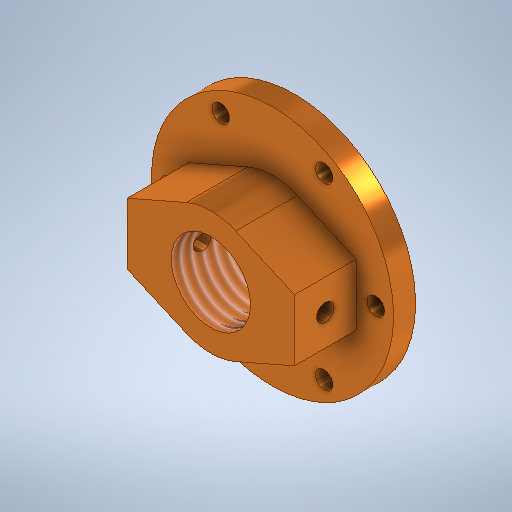
# Autodesk Inventor part: 109
Saved by Autodesk Inventor 2025.1 (Build 291241000, 241)
## iProperties
Created: 2024-06-07
Part Number: 109
Material: Gold
Document SubType Name: Modeling
Designer: ffogue
Density: 19.3 g/cm^3
Appearance: Metall - 1600F (heiß)
Author: ffogue
Autodesk Inventor part; units mm, degrees
ref_plane "YZ Plane" through (0, 0, 0) normal (1, 0, 0) x (0, 1, 0)
ref_plane "XZ Plane" through (0, 0, 0) normal (0, 1, 0) x (-1, 0, 0)
ref_plane "XY Plane" through (0, 0, 0) normal (0, 0, 1) x (1, 0, 0)
sketch "Skizze1" plane through (0, 0, 0) normal (0, 1, 0) x (-1, 0, 0)
  circle A0 centre (0, 0) radius 27.5
  dimension "d0" = 55
  constraints: 1 centre point, 1 coincident
  measures "d0" diameter of A0
extrude "Extrusion1" add sketch "Skizze1" along normal blind 5
sketch "Skizze2" plane through (0, 5, 0) normal (0, 1, 0) x (1, 0, 0)
  circle A0 centre (0, 0) radius 15
  dimension "d4" = 30
  constraints: 1 centre point, 1 coincident
  measures "d4" diameter of A0
extrude "Extrusion2" add sketch "Skizze2" along normal blind 1.5
sketch "Skizze3" plane through (0, 6.5, 0) normal (0, 1, 0) x (1, 0, 0)
  circle A0 centre (0, 0) radius 15 projected
  line L0 (-6.5, 13.5185) -> (-6.5, 12)
  line L1 (-4.5, 10) -> (4.5, 10)
  line L2 (6.5, 12) -> (6.5, 13.5185)
  line L3 (0, -15) -> (0, 15) construction
  arc A1 (-6.5, 12) -> (-4.5, 10) centre (-4.5, 12) ccw
  arc A2 (4.5, 10) -> (6.5, 12) centre (4.5, 12) ccw
  point P0 (-6.5, 10)
  point P1 (6.5, 10)
  dimension "d7" = 13
  dimension "d8" = 10
  dimension "d9" = 2
  constraints: 8 end point, 8 point on circle, 4 point on line, 4 tangent, 2 centre point, 2 perpendicular, 2 vertical, 1 equal radius, 1 horizontal alignment, 1 midpoint, 1 other
  measures "d7" distance of point (-6.5, 10) point (6.5, 10)
  measures "d8" distance from line of L1 point (0, 0)
  measures "d9" radius of A1
extrude "Extrusion3" cut sketch "Skizze3" against normal blind 1.5 contours L2 A2 L1 A1 L0 A0 picked at (0, 11.6667)
sketch "Skizze4" plane through (0, 5, 0) normal (0, 1, 0) x (1, 0, 0)
  circle A0 centre (0, 0) radius 23.5 construction
  point P0 (-23.5, 0)
  dimension "d12" = 47
  constraints: 2 horizontal alignment, 1 coincident, 2 other
hole "Bohrung1" at (-23.5, 5, 0) direction (0, -1, 0) diameter 4 end through all
pattern_circular "Runde Anordnung1" count 6 over 360 about axis through (0, 0, 0) along (0, 1, 0) of "Bohrung1"
sketch "Skizze5" plane through (0, 0, 0) normal (0, -1, 0) x (1, 0, 0)
  line L0 (-19, -7) -> (-19, 7)
  line L1 (-19, 7) -> (-5.6144, 12.8489)
  line L2 (-19, -7) -> (-5.6144, -12.8489)
  line L3 (5.6144, -12.8489) -> (19, -7)
  line L4 (19, -7) -> (19, 7)
  line L5 (19, 7) -> (5.6144, 12.8489)
  line L6 (0, -28.3232) -> (0, 28.3232) construction
  arc A0 (-5.6144, -12.8489) -> (5.6144, -12.8489) centre (0, 0) ccw
  arc A1 (5.6144, 12.8489) -> (-5.6144, 12.8489) centre (0, 0) ccw
  point P0 (-19, 0)
  point P1 (19, 0)
  dimension "d27" = 14
  dimension "d28" = 14
  dimension "d29" = 38
  constraints: 14 end point, 4 point on circle, 4 tangent, 3 midpoint, 3 vertical, 2 centre point, 2 coincident, 2 horizontal alignment, 1 vertical alignment, 1 other
  measures "d27" distance of L0.start L0.end
  measures "d28" distance of L3.end L4.end
  measures "d29" distance between parallel lines of L4 L0
extrude "Extrusion4" add sketch "Skizze5" along normal blind 14
sketch "Skizze6" plane through (0, -14, 0) normal (0, -1, 0) x (1, 0, 0)
  circle A0 centre (0, 0) radius 9
  dimension "d32" = 18
  constraints: 1 centre point, 1 coincident
  measures "d32" diameter of A0
extrude "Extrusion5" cut sketch "Skizze6" against normal blind 15.5
thread "Gewinde1" size "M18x2.5" class "6H" standard "ISO Metric profile" length 14
sketch "Skizze7" plane through (-19, 0, -7) normal (-1, 0, 0) x (0, 0, 1)
  line L0 (-5.8489, 0) -> (-5.8489, -14) projected
  line L1 (0, 0) -> (14, 0) projected
  point P0 (7, 0)
  point P1 (7, -7)
  point P2 (-5.8489, -7)
  point P3 (7, 0)
  constraints: 2 midpoint, 1 horizontal alignment, 1 vertical alignment
hole "Bohrung2" at (-19, -7, 0) direction (1, 0, 0) diameter 4 depth 10 tip angle 118
mirror "Mirror1" about plane through (0, 0, 0) normal (1, 0, 0) of "Bohrung2"
